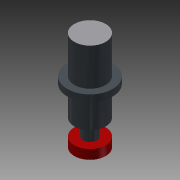
# Autodesk Inventor part: licht_taster
Saved by Autodesk Inventor 2016 SP2 (Build 200236200, 236)
## iProperties
Created: 2018-01-12
Part Number: licht_taster
Material: Generisch
Document SubType Name: Modeling
Designer: wepet
Density: 1 g/cm^3
Appearance: Vorgabe
Mass: 0.702879 g
Surface Area: 6.22915 cm^2
Volume: 0.702879 cm^3
Author: wepet
Autodesk Inventor part; units mm, degrees
ref_plane "YZ Plane" through (0, 0, 0) normal (1, 0, 0) x (0, 1, 0)
ref_plane "XZ Plane" through (0, 0, 0) normal (0, 1, 0) x (-1, 0, 0)
ref_plane "XY Plane" through (0, 0, 0) normal (0, 0, 1) x (1, 0, 0)
sketch "Skizze1" plane through (0, 0, 0) normal (0, 1, 0) x (-1, 0, 0)
  line L0 (0, 0) -> (3.35, 0)
  line L1 (3.35, 0) -> (3.35, -8)
  line L2 (3.35, -8) -> (4.85, -8)
  line L3 (4.85, -8) -> (4.85, -9.4)
  line L4 (4.85, -9.4) -> (3.35, -9.4)
  line L5 (3.35, -9.4) -> (3.35, -15.7)
  line L6 (3.35, -15.7) -> (1.5, -15.7)
  line L7 (1.5, -15.7) -> (1.5, -19.2)
  line L8 (1.5, -19.2) -> (3.35, -19.2)
  line L9 (3.35, -19.2) -> (3.35, -21.2)
  line L10 (3.35, -21.2) -> (0, -21.2)
  line L11 (0, 0) -> (0, -21.2)
  dimension "d0" = 3.35
  dimension "d1" = 8
  dimension "d3" = 5.5
  dimension "d4" = 11.8
  dimension "d5" = 21.2
  dimension "d6" = 2
  dimension "d7" = 1.5
  dimension "d10" = 4.85
  constraints: 24 end point, 9 perpendicular, 2 point on line, 1 collinear, 1 horizontal, 1 vertical
  measures "d0" distance of L0.start L0.end
  measures "d1" distance of L0.end L1.end
  measures "d3" distance between parallel lines of L6 L10
  measures "d4" distance between parallel lines of L4 L10
  measures "d5" distance between parallel lines of L0 L10
  measures "d6" distance between parallel lines of L10 L8
  measures "d7" distance from line of L0.start L7
  measures "d10" distance from line of L0.start L3
revolve "Umdrehung1" add sketch "Skizze1" angle 360 about axis through (0, 0, 0) along (0, 0, -1)
